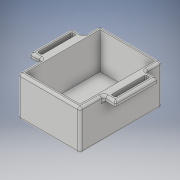
# Autodesk Inventor part: wrist box
Saved by Autodesk Inventor 2017 (Build 210142000, 142)
## iProperties
Created: 2018-06-23
Part Number: wrist box
Material: Generic
Document SubType Name: Modeling
Designer: Mitch
Density: 1 g/cm^3
Appearance: Default
Author: Mitch
Autodesk Inventor part; units mm, degrees
ref_plane "YZ Plane" through (0, 0, 0) normal (1, 0, 0) x (0, 1, 0)
ref_plane "XZ Plane" through (0, 0, 0) normal (0, 1, 0) x (-1, 0, 0)
ref_plane "XY Plane" through (0, 0, 0) normal (0, 0, 1) x (1, 0, 0)
sketch "Sketch1" plane through (0, 0, 0) normal (0, 1, 0) x (-1, 0, 0)
  line L0 (0, 0) -> (43.18, 0)
  line L1 (43.18, 0) -> (43.18, -57.15)
  line L2 (43.18, -57.15) -> (0, -57.15)
  line L3 (0, -57.15) -> (0, 0)
  dimension "d0" = 43.18
  dimension "d1" = 57.15
  constraints: 8 end point, 2 parallel, 1 horizontal, 1 perpendicular
  measures "d0" distance of L1.end L2.end
  measures "d1" distance of L0.end L1.end
extrude "Extrusion1" add sketch "Sketch1" along normal blind 27.94
shell "Shell1" thickness 2.54 removed faces 1 at (-14.3933, 27.94, -19.05)
sketch "Sketch2" plane through (0, 27.94, 0) normal (0, 1, 0) x (1, 0, 0)
  line L0 (0, 0) -> (0, 57.15) projected
  line L1 (0, 45.72) -> (8.255, 45.72)
  line L2 (8.255, 45.72) -> (8.255, 16.51)
  line L3 (8.255, 16.51) -> (0, 16.51)
  line L4 (0, 16.51) -> (0, 45.72)
  line L5 (-43.18, 57.15) -> (-43.18, 0) projected
  line L6 (-43.18, 45.72) -> (-51.435, 45.72)
  line L7 (-51.435, 45.72) -> (-51.435, 16.51)
  line L8 (-51.435, 16.51) -> (-43.18, 16.51)
  line L9 (-43.18, 16.51) -> (-43.18, 45.72)
  line L10 (0, 57.15) -> (-43.18, 57.15) projected
  line L11 (-48.895, 19.05) -> (-48.895, 43.18)
  line L12 (-48.895, 43.18) -> (-45.72, 43.18)
  line L13 (-45.72, 43.18) -> (-45.72, 19.05)
  line L14 (-45.72, 19.05) -> (-48.895, 19.05)
  line L15 (5.715, 19.05) -> (5.715, 43.18)
  line L16 (5.715, 43.18) -> (2.54, 43.18)
  line L17 (2.54, 43.18) -> (2.54, 19.05)
  line L18 (2.54, 19.05) -> (5.715, 19.05)
  dimension "d5" = 11.43
  dimension "d6" = 29.21
  dimension "d7" = 8.255
  dimension "d8" = 8.255
  dimension "d9" = 2.54
  dimension "d10" = 2.54
  constraints: 32 end point, 8 parallel, 4 perpendicular, 4 point on line, 2 horizontal, 6 other
  measures "d5" distance between parallel lines of L6 L10
  measures "d6" distance between parallel lines of L8 L6
  measures "d7" distance between parallel lines of L7 L5
  measures "d8" distance between parallel lines of L0 L2
  measures "d9" distance between parallel lines of L7 L11
  measures "d10" distance between parallel lines of L2 L15
extrude "Extrusion2" add sketch "Sketch2" against normal blind 3.175
fillet "Fillet1" radius 1.5875 6 edges at (-43.18, 24.765, -31.115) (-43.18, 26.3525, -45.72) (-43.18, 26.3525, -16.51) (0, 24.765, -31.115) (0, 26.3525, -16.51) (0, 26.3525, -45.72)
fillet "Fillet2" radius 0.7937 12 edges at (2.54, 26.3525, -43.18) (5.715, 26.3525, -43.18) (2.54, 26.3525, -19.05) (5.715, 26.3525, -19.05) (-45.72, 26.3525, -19.05) (-45.72, 26.3525, -43.18) (-48.895, 26.3525, -43.18) (-48.895, 26.3525, -19.05) (-51.435, 26.3525, -16.51) (-51.435, 26.3525, -45.72) (8.255, 26.3525, -16.51) (8.255, 26.3525, -45.72)
fillet "Fillet3" radius 1.5875 4 edges at (-43.18, 0, -28.575) (-21.59, 0, 0) (0, 0, -28.575) (-21.59, 0, -57.15)
fillet "Fillet4" radius 1.5875 28 edges at (-0.465, 0.465, -0.465) (0, 14.7638, 0) (-42.715, 0.465, -0.465) (-43.18, 14.7638, 0) (-0.465, 0.465, -56.685) (0, 14.7638, -57.15) (-42.715, 0.465, -56.685) (-43.18, 14.7638, -57.15) (-21.59, 27.94, -57.15) (-21.59, 27.94, 0) (-43.645, 27.94, -16.045) (-47.7044, 27.94, -16.51) (-51.2025, 27.94, -16.7425) (-51.435, 27.94, -31.115) (-51.2025, 27.94, -45.4875) (-47.7044, 27.94, -45.72) (-43.645, 27.94, -46.185) (-43.18, 27.94, -52.2288) (-43.18, 27.94, -7.4613) (0.465, 27.94, -16.045) (4.5244, 27.94, -16.51) (8.0225, 27.94, -16.7425) (8.255, 27.94, -31.115) (8.0225, 27.94, -45.4875) (4.5244, 27.94, -45.72) (0.465, 27.94, -46.185) (0, 27.94, -52.2288) (0, 27.94, -7.4613)
body "Solid1"
